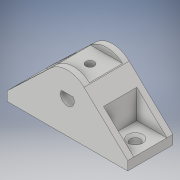
# Autodesk Inventor part: engine_center
Saved by Autodesk Inventor 2019.4 (Build 234330000, 330)
## iProperties
Created: 2020-04-09
Part Number: engine_center
Material: Типовые
Document SubType Name: Modeling
Designer: NoName
Density: 1 g/cm^3
Appearance: По умолчанию
Author: NoName
Autodesk Inventor part; units mm, degrees
ref_plane "YZ Plane" through (0, 0, 0) normal (1, 0, 0) x (0, 1, 0)
sketch "Эскиз1" plane through (0, 0, 0) normal (0, 0, 1) x (1, 0, 0)
  line L0 (-20, 0) -> (20, 0)
  line L1 (20, 0) -> (20, 3)
  line L2 (20, 3) -> (5.5172, 16.7931)
  line L3 (0, 0) -> (0, 19)
  line L4 (-20, 0) -> (-20, 3)
  line L5 (-20, 3) -> (-5.5172, 16.7931)
  arc A0 (5.5172, 16.7931) -> (-5.5172, 16.7931) centre (0, 11) ccw
  dimension "d0" = 40
  dimension "d1" = 3
  dimension "d2" = 8
  dimension "d3" = 11
  constraints: 12 end point, 3 point on circle, 2 symmetric about line, 1 centre point, 1 coincident, 1 horizontal, 1 midpoint, 1 perpendicular, 1 point on line, 1 tangent, 1 vertical
  measures "d0" distance of L0.start L0.end
  measures "d1" distance of L0.end L1.end
  measures "d2" radius of A0
  measures "d3" distance from line of L0 A0.centre
extrude "Выдавливание1" add sketch "Эскиз1" along normal blind 15
ref_plane "РабПлоскость1" through (20, 3, 15) normal (0, -1, 0) x (1, 0, 0)
sketch "Эскиз2" plane through (20, 3, 15) normal (0, -1, 0) x (1, 0, 0)
  line L0 (-40, -15) -> (-40, 0) projected
  line L1 (-40, -13) -> (-30, -13)
  line L2 (-30, -13) -> (-30, -2)
  line L3 (-30, -2) -> (-40, -2)
  line L4 (-40, -2) -> (-40, -13)
  line L5 (0, -15) -> (0, 0) projected
  line L6 (0, -13) -> (-10, -13)
  line L7 (-10, -13) -> (-10, -2)
  line L8 (-10, -2) -> (0, -2)
  line L9 (0, -2) -> (0, -13)
  line L10 (-40, -7.5) -> (0, -7.5)
  line L11 (-20, -15) -> (-20, 0)
  line L12 (-40, 0) -> (0, 0) projected
  point P0 (-10, -7.5)
  point P1 (-30, -7.5)
  point P2 (-40, -7.5)
  dimension "d6" = 20
  dimension "d7" = 11
  constraints: 20 end point, 8 midpoint, 4 parallel, 4 point on line, 2 horizontal, 2 perpendicular, 1 horizontal alignment, 1 other
  measures "d6" distance between parallel lines of L2 L7
  measures "d7" distance between parallel lines of L8 L6
extrude "Выдавливание2" cut sketch "Эскиз2" against normal through all contours L0 L10 L2 L1 | L0 L3 L2 L10 | L10 L5 L6 L7 | L7 L8 L5 L10
sketch "Эскиз3" plane through (20, 3, 15) normal (0, 1, 0) x (1, 0, 0)
  line L0 (-40, 13) -> (-40, 2) projected
  line L1 (-20, 15) -> (-20, 0)
  line L2 (-40, 0) -> (0, 0) projected
  point P0 (-35, 7.5)
  point P1 (-5, 7.5)
  point P2 (-40, 7.5)
  dimension "d17" = 30
  constraints: 2 end point, 2 horizontal alignment, 2 midpoint, 1 symmetric about line
  measures "d17" distance of point (-35, 7.5) point (-5, 7.5)
hole "Отверстие1" at (-15, 3, 7.5) at (15, 3, 7.5) direction (0, -1, 0) diameter 3.3 end through all countersink diameter 5 countersink angle 90
ref_plane "РабПлоскость2" through (-20, 17, 0) normal (0, -1, 0) x (1, 0, 0)
sketch "Эскиз5" plane through (-20, 17, 0) normal (0, -1, 0) x (1, 0, 0)
  line L0 (0, 2) -> (10, 2) projected
  line L1 (30, 13) -> (30, 2) projected
  line L2 (10, 2) -> (30, 2)
  line L3 (30, 2) -> (30, 13)
  line L4 (30, 13) -> (10, 13)
  line L5 (10, 13) -> (10, 2)
  point P0 (20, 0)
  constraints: 8 end point, 2 parallel, 1 horizontal, 1 perpendicular
extrude "Выдавливание3" cut sketch "Эскиз5" against normal through all
sketch "Эскиз6" plane through (0, 0, 15) normal (0, 0, 1) x (1, 0, 0)
  arc A0 (5.5172, 16.7931) -> (-5.5172, 16.7931) centre (0, 11) ccw projected
  arc A1 (-1.9621, 12.2) -> (1.9621, 12.2) centre (0, 11) ccw
  line L0 (-1.9621, 12.2) -> (1.9621, 12.2)
  point P0 (0, 0)
  dimension "d32" = 2.3
  dimension "d33" = 1.2
  constraints: 2 end point, 2 point on circle, 1 centre point, 1 coincident, 1 horizontal, 1 horizontal alignment
  measures "d32" radius of A1
  measures "d33" distance from line of A0.centre L0
extrude "Выдавливание4" cut sketch "Эскиз6" against normal through all
sketch "Эскиз7" plane through (-20, 17, 0) normal (0, 1, 0) x (1, 0, 0)
  line L0 (14.7085, -13) -> (14.7085, -2) projected
  line L1 (14.7085, -13) -> (25.2915, -13) projected
  point P0 (20, 0)
  point P1 (20, -7.5)
  point P2 (14.7085, -7.5)
  point P3 (20, -13)
  constraints: 2 midpoint, 1 horizontal alignment, 1 vertical alignment
hole "Отверстие3" at (0, 17, 7.5) direction (0, -1, 0) diameter 2.8 depth 4.8
